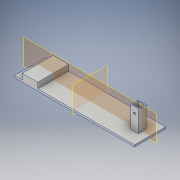
# Autodesk Inventor part: SupportPlateToAttachToRobotBase
Saved by Autodesk Inventor 2016 SP1 (Build 200210100, 210)
## iProperties
Created: 2016-02-07
Part Number: SupportPlateToAttachToRobotBase
Material: Aluminum 6061
Document SubType Name: Modeling
Designer: steele
Density: 2.7 g/cm^3
Appearance: Aluminum - Flat
Author: steele
Autodesk Inventor part; units mm, degrees
ref_plane "XZ Plane" through (0, 0, 0) normal (0, 1, 0) x (-1, 0, 0)
sketch "Sketch1" plane through (0, 0, 0) normal (0, 1, 0) x (-1, 0, 0)
  line L0 (196.85, 50.8) -> (-196.85, 50.8)
  line L1 (-196.85, 50.8) -> (-196.85, -50.8)
  line L2 (-196.85, -50.8) -> (196.85, -50.8)
  line L3 (196.85, -50.8) -> (196.85, 50.8)
  line L4 (196.85, 50.8) -> (-196.85, -50.8) construction
  line L5 (-196.85, 50.8) -> (196.85, -50.8) construction
  point P0 (0, 0)
  dimension "d0" = 101.6
  dimension "d1" = 393.7
  constraints: 12 end point, 2 midpoint, 2 parallel, 1 horizontal, 1 perpendicular
  measures "d0" distance of L2.end L0.start
  measures "d1" distance of L0.start L0.end
extrude "Extrusion1" add sketch "Sketch1" along normal blind 6.35
sketch "Sketch2" plane through (0, 6.35, 0) normal (0, 1, 0) x (1, 0, 0)
  line L0 (146.05, -12.7) -> (171.45, -12.7)
  line L1 (171.45, -12.7) -> (171.45, 12.7)
  line L2 (171.45, 12.7) -> (146.05, 12.7)
  line L3 (146.05, 12.7) -> (146.05, -12.7)
  line L4 (146.05, -12.7) -> (171.45, 12.7) construction
  line L5 (171.45, -12.7) -> (146.05, 12.7) construction
  line L6 (149.225, -9.525) -> (168.275, -9.525)
  line L7 (168.275, -9.525) -> (168.275, 9.525)
  line L8 (168.275, 9.525) -> (149.225, 9.525)
  line L9 (149.225, 9.525) -> (149.225, -9.525)
  line L10 (149.225, -9.525) -> (168.275, 9.525) construction
  line L11 (168.275, -9.525) -> (149.225, 9.525) construction
  line L12 (196.85, -50.8) -> (196.85, 50.8) projected
  line L13 (-196.85, -50.8) -> (196.85, -50.8) projected
  point P0 (0, 0)
  point P1 (158.75, 0)
  dimension "d4" = 25.4
  dimension "d5" = 25.4
  dimension "d6" = 3.175
  dimension "d7" = 3.175
  dimension "d8" = 25.4
  dimension "d14" = 38.1
  constraints: 24 end point, 4 midpoint, 4 parallel, 2 horizontal, 2 perpendicular
  measures "d4" distance of L0.end L1.end
  measures "d5" distance of L1.end L2.end
  measures "d6" distance between parallel lines of L6 L0
  measures "d7" distance between parallel lines of L9 L3
  measures "d8" distance between parallel lines of L1 L12
  measures "d14" distance between parallel lines of L0 L13
extrude "Extrusion2" add sketch "Sketch2" along normal blind 69.7992
sketch "Sketch3" plane through (171.45, 6.35, 12.7) normal (1, 0, 0) x (0, 0, -1)
  line L0 (0, 69.7992) -> (25.4, 69.7992) projected
  circle A0 centre (12.7, 69.7992) radius 4.7625
  point P0 (12.7, -6.35)
  dimension "d11" = 9.525
  constraints: 1 centre point, 1 midpoint
  measures "d11" diameter of A0
extrude "Extrusion3" cut sketch "Sketch3" against normal through all
sketch "Sketch4" plane through (0, 6.35, 0) normal (0, 1, 0) x (1, 0, 0)
  line L0 (-171.45, -50.8) -> (-120.65, -50.8)
  line L1 (-120.65, -50.8) -> (-120.65, 50.8)
  line L2 (-120.65, 50.8) -> (-171.45, 50.8)
  line L3 (-171.45, 50.8) -> (-171.45, -50.8)
  line L4 (-171.45, -50.8) -> (-120.65, 50.8) construction
  line L5 (-120.65, -50.8) -> (-171.45, 50.8) construction
  line L6 (-196.85, 50.8) -> (-196.85, -50.8) projected
  line L7 (-196.85, -50.8) -> (196.85, -50.8) projected
  point P0 (0, 0)
  point P1 (-146.05, 0)
  dimension "d15" = 50.8
  dimension "d16" = 25.4
  dimension "d17" = 101.6
  constraints: 12 end point, 2 midpoint, 2 parallel, 1 collinear, 1 horizontal, 1 perpendicular
  measures "d15" distance of L1.end L2.end
  measures "d16" distance between parallel lines of L3 L6
  measures "d17" distance of L2.end L0.start
extrude "Extrusion4" add sketch "Sketch4" along normal blind 18.9992
sketch "Sketch5" plane through (0, 6.35, 0) normal (0, 1, 0) x (1, 0, 0)
  line L0 (196.85, 50.8) -> (-196.85, 50.8) projected
  line L1 (-101.6, 50.8) -> (101.6, 50.8)
  line L2 (101.6, 50.8) -> (101.6, 25.4)
  line L3 (101.6, 25.4) -> (-101.6, 25.4)
  line L4 (-101.6, 25.4) -> (-101.6, 50.8)
  point P0 (0, 0)
  dimension "d20" = 101.6
  dimension "d21" = 101.6
  dimension "d22" = 25.4
  constraints: 8 end point, 2 parallel, 1 horizontal, 1 perpendicular, 1 point on line
  measures "d20" distance from line of point (0, 0) L4
  measures "d21" distance from line of point (0, 0) L2
  measures "d22" distance of L1.end L2.end
sketch "Sketch7" plane through (0, 6.35, 0) normal (0, 1, 0) x (1, 0, 0)
  line L0 (-196.85, -50.8) -> (196.85, -50.8) projected
  line L1 (-101.6, -50.8) -> (101.6, -50.8)
  line L2 (101.6, -50.8) -> (101.6, 0)
  line L3 (101.6, 0) -> (-101.6, 0)
  line L4 (-101.6, 0) -> (-101.6, -50.8)
  line L5 (-101.6, 25.4) -> (-101.6, 50.8) projected
  line L6 (101.6, 50.8) -> (101.6, 25.4) projected
  line L7 (101.6, 25.4) -> (-101.6, 25.4) projected
  point P0 (0, 0)
  dimension "d28" = 25.4
  constraints: 8 end point, 2 collinear, 2 parallel, 1 horizontal, 1 perpendicular, 1 point on line
  measures "d28" distance between parallel lines of L3 L7
equation "\"d0\" = width"
equation "\"d1\" = length"
equation "\"d2\" = thickness"
equation "\"width\" = 101.6"
equation "\"length\" = 393.7"
equation "\"thickness\" = 6.35"
body "Solid1"
